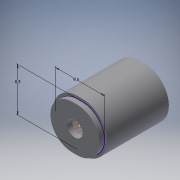
# Autodesk Inventor part: chamber_10mm
Saved by Autodesk Inventor 2016 (Build 200138000, 138)
## iProperties
Created: 2016-08-11
Part Number: chamber_10mm
Material: Generic
Document SubType Name: Modeling
Designer: GentnerLab
Density: 1 g/cm^3
Appearance: Default
Author: GentnerLab
Autodesk Inventor part; units mm, degrees
ref_plane "YZ Plane" through (0, 0, 0) normal (1, 0, 0) x (0, 1, 0)
ref_plane "XZ Plane" through (0, 0, 0) normal (0, 1, 0) x (-1, 0, 0)
ref_plane "XY Plane" through (0, 0, 0) normal (0, 0, 1) x (1, 0, 0)
sketch "Sketch1" plane through (0, 0, 0) normal (0, 1, 0) x (-1, 0, 0)
  line L0 (-0.5, 0) -> (0.5, 0) construction
  line L1 (-0.5, -4.25) -> (0.5, -4.25)
  line L2 (0.5, 4.25) -> (-0.5, 4.25)
  arc A0 (-0.5, 4.25) -> (-0.5, -4.25) centre (-0.5, 0) ccw
  arc A1 (0.5, -4.25) -> (0.5, 4.25) centre (0.5, 0) ccw
  point P0 (0, 0)
  point P1 (0, 0)
  dimension "d2" = 8.5
  dimension "d3" = 9.5
  constraints: 8 end point, 4 point on circle, 4 tangent, 2 centre point, 1 coincident, 1 horizontal, 1 midpoint, 1 parallel
  measures "d2" distance between parallel lines of L1 L2
surface extrude "ExtrusionSrf1" sketch "Sketch1" along normal blind 12 shown yes curves L1 A1 L2 A0
extrude "Extrusion1" add sketch "Sketch1" against normal blind 1
hole "Hole1" at (0, 0, 0) direction (0, -1, 0) diameter 3 end through all
thicken "Thicken1" operation add thickness 0.5 both sides no extend neighbours no toward (-0.5344658, 0, 0.8451901) faces at (-2.7715, 8, 3.5921) (0.1667, 4, -4.25) (1.1817, 8, -4.195) (-0.1667, 4, 4.25)
sketch "Sketch2" plane through (0.5, 0, -4.75) normal (0, 0, -1) x (-1, 0, 0)
  point P0 (0.5, 0)
sketch "Sketch3" plane through (0.5, 0, -4.75) normal (0, 0, -1) x (-1, 0, 0)
  point P0 (0.5, 0)
sketch "Sketch4" plane through (0.5, 0, -4.75) normal (0, 0, -1) x (-1, 0, 0)
  line L0 (0.5, 0) -> (0.5, 12)
  line L1 (0, 12) -> (1, 12) projected
  line L2 (-0.5, 10.5) -> (1.5, 10.5)
  line L3 (1.5, 10.5) -> (1.5, 12)
  line L4 (1.5, 12) -> (-0.5, 12)
  line L5 (-0.5, 12) -> (-0.5, 10.5)
  point P0 (0.5, 11.1306)
  dimension "d17" = 2
  dimension "d18" = 1
  dimension "d19" = 0
  dimension "d20" = 1.5
  constraints: 10 end point, 2 parallel, 1 horizontal, 1 midpoint, 1 perpendicular, 1 point on line
  measures "d17" distance between parallel lines of L5 L3
  measures "d18" distance between parallel lines of L0 L5
  measures "d19" distance between parallel lines of L1 L4
  measures "d20" distance from line of L0.end L2
extrude "Extrusion2" cut sketch "Sketch4" against normal up to surface (4.75 mm away)
equation "\"d18\" = 0.5 * d17"
body "Solid1"
body "Srf1"
